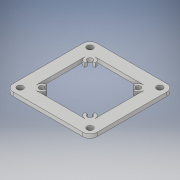
# Autodesk Inventor part: CameraMount
Saved by Autodesk Inventor 2018 (Build 220112000, 112)
## iProperties
Created: 2019-10-01
Part Number: CameraMount
Material: Generic
Document SubType Name: Modeling
Designer: anirudh
Density: 1 g/cm^3
Appearance: Default
Author: anirudh
Autodesk Inventor part; units mm, degrees
ref_plane "YZ Plane" through (0, 0, 0) normal (1, 0, 0) x (0, 1, 0)
ref_plane "XZ Plane" through (0, 0, 0) normal (0, 1, 0) x (-1, 0, 0)
ref_plane "XY Plane" through (0, 0, 0) normal (0, 0, 1) x (1, 0, 0)
sketch "Sketch1" plane through (0, 0, 0) normal (0, 1, 0) x (-1, 0, 0)
  arc A0 (-101.3954, 102.8954) -> (-102.8954, 101.3954) centre (-102.8954, 102.8954) ccw
  arc A1 (-101.3954, 102.8954) -> (-102.8954, 101.3954) centre (-102.8954, 102.8954) ccw
  arc A2 (-102.8954, 76.4046) -> (-101.3954, 74.9046) centre (-102.8954, 74.9046) ccw
  arc A3 (-102.8954, 76.4046) -> (-101.3954, 74.9046) centre (-102.8954, 74.9046) ccw
  arc A4 (-76.4046, 74.9046) -> (-74.9046, 76.4046) centre (-74.9046, 74.9046) ccw
  arc A5 (-76.4046, 74.9046) -> (-74.9046, 76.4046) centre (-74.9046, 74.9046) ccw
  arc A6 (-74.9046, 101.3954) -> (-76.4046, 102.8954) centre (-74.9046, 102.8954) ccw
  arc A7 (-74.9046, 101.3954) -> (-76.4046, 102.8954) centre (-74.9046, 102.8954) ccw
  arc A8 (-105.9, 102.8954) -> (-102.8954, 99.8908) centre (-102.8954, 102.8954) ccw
  arc A9 (-102.8954, 77.9092) -> (-105.9, 74.9046) centre (-102.8954, 74.9046) ccw
  line L0 (-102.8954, 77.9092) -> (-102.8954, 76.4046)
  line L1 (-74.9046, 76.4046) -> (-74.9046, 77.9092)
  line L2 (-74.9046, 99.8908) -> (-74.9046, 101.3954)
  line L3 (-105.9, 74.9046) -> (-105.9, 102.8954)
  arc A10 (-99.8908, 102.8954) -> (-102.8954, 105.9) centre (-102.8954, 102.8954) ccw
  line L4 (-102.8954, 105.9) -> (-74.9046, 105.9)
  line L5 (-74.9046, 71.9) -> (-102.8954, 71.9)
  line L6 (-102.8954, 71.9) -> (-74.9046, 71.9)
  arc A11 (-71.9, 74.9046) -> (-74.9046, 77.9092) centre (-74.9046, 74.9046) ccw
  line L7 (-71.9, 74.9046) -> (-71.9, 102.8954)
  line L8 (-77.9092, 102.8954) -> (-76.4046, 102.8954)
  line L9 (-76.4046, 102.8954) -> (-77.9092, 102.8954)
  line L10 (-74.9046, 101.3954) -> (-74.9046, 99.8908)
  line L11 (-77.9092, 74.9046) -> (-76.4046, 74.9046)
  line L12 (-77.9092, 74.9046) -> (-76.4046, 74.9046)
  line L13 (-74.9046, 76.4046) -> (-74.9046, 77.9092)
  line L14 (-101.3954, 74.9046) -> (-99.8908, 74.9046)
  line L15 (-101.3954, 74.9046) -> (-99.8908, 74.9046)
  line L16 (-102.8954, 76.4046) -> (-102.8954, 77.9092)
  line L17 (-102.8954, 101.3954) -> (-102.8954, 99.8908)
  line L18 (-102.8954, 99.8908) -> (-102.8954, 101.3954)
  line L19 (-101.3954, 102.8954) -> (-99.8908, 102.8954)
  arc A12 (-74.9046, 99.8908) -> (-71.9, 102.8954) centre (-74.9046, 102.8954) ccw
  arc A13 (-74.9046, 105.9) -> (-77.9092, 102.8954) centre (-74.9046, 102.8954) ccw
  arc A14 (-99.8908, 102.8954) -> (-102.8954, 105.9) centre (-102.8954, 102.8954) ccw
  arc A15 (-105.9, 102.8954) -> (-102.8954, 99.8908) centre (-102.8954, 102.8954) ccw
  arc A16 (-102.8954, 77.9092) -> (-105.9, 74.9046) centre (-102.8954, 74.9046) ccw
  arc A17 (-102.8954, 71.9) -> (-99.8908, 74.9046) centre (-102.8954, 74.9046) ccw
  arc A18 (-77.9092, 74.9046) -> (-74.9046, 71.9) centre (-74.9046, 74.9046) ccw
  arc A19 (-71.9, 74.9046) -> (-74.9046, 77.9092) centre (-74.9046, 74.9046) ccw
  line L20 (-102.8954, 74.9046) -> (-90.1954, 74.9046) construction
  line L21 (-102.8954, 74.9046) -> (-94.0054, 74.9046) construction
  circle A20 centre (-109.1816, 68.6184) radius 1.75
  circle A21 centre (-109.1816, 109.1816) radius 1.75
  circle A22 centre (-68.6184, 68.6184) radius 1.75
  circle A23 centre (-68.6184, 109.1816) radius 1.75
  arc A24 (-113.3091, 68.6184) -> (-109.1816, 64.4909) centre (-109.1816, 68.6184) ccw
  arc A25 (-68.6184, 64.4909) -> (-64.4909, 68.6184) centre (-68.6184, 68.6184) ccw
  arc A26 (-109.1816, 113.3091) -> (-113.3091, 109.1816) centre (-109.1816, 109.1816) ccw
  arc A27 (-64.4909, 109.1816) -> (-68.6184, 113.3091) centre (-68.6184, 109.1816) ccw
  line L22 (-109.1816, 64.4909) -> (-68.6184, 64.4909)
  line L23 (-64.4909, 68.6184) -> (-64.4909, 109.1816)
  line L24 (-113.3091, 68.6184) -> (-113.3091, 109.1816)
  line L25 (-109.1816, 113.3091) -> (-68.6184, 113.3091)
  point P0 (0, 0)
  point P1 (-88.9, 127)
  dimension "d0" = 8.255
  constraints: 52 end point, 48 point on circle, 28 centre point, 12 coincident, 9 tangent, 6 equal length, 6 horizontal, 3 perpendicular, 3 vertical
  measures "d0" diameter of A24
extrude "Extrusion1" add sketch "Sketch1" along normal blind 2.286
body "Solid1"
